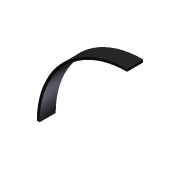
# Autodesk Inventor part: Frame_FrontConveyorGuideCurve
Saved by Autodesk Inventor 2012 (Build 160160000, 160)
## iProperties
Created: 2012-01-25
Part Number: Frame_FrontConveyorGuideCurve
Material: Aluminum-6061
Document SubType Name: Modeling
Designer: JesseK
Mass: 219.082 g
Surface Area: 301.896 cm^2
Volume: 80.842 cm^3
Density: 2.71 g/cm^3
Author: JesseK
Autodesk Inventor part; units mm, degrees
ref_plane "YZ Plane" through (0, 0, 0) normal (1, 0, 0) x (0, 1, 0)
ref_plane "XZ Plane" through (0, 0, 0) normal (0, 1, 0) x (-1, 0, 0)
ref_plane "XY Plane" through (0, 0, 0) normal (0, 0, 1) x (1, 0, 0)
sketch "Sketch1" plane through (0, 0, 0) normal (0, 0, 1) x (1, 0, 0)
  arc A0 (0, 209.55) -> (-209.55, 0) centre (0, 0) ccw
  arc A1 (0, 215.9) -> (-215.9, 0) centre (0, 0) ccw
  line L0 (0, 215.9) -> (0, 209.55)
  line L1 (-215.9, 0) -> (-209.55, 0)
  dimension "d0" = 209.55
  dimension "d1" = 6.35
  constraints: 4 end point, 4 point on circle, 2 centre point, 2 coincident, 1 horizontal, 1 vertical
  measures "d0" radius of A0
  measures "d1" radial gap between concentric circles of A0 A1
extrude "Extrusion1" add sketch "Sketch1" along normal blind 38.1
body "Solid1"
